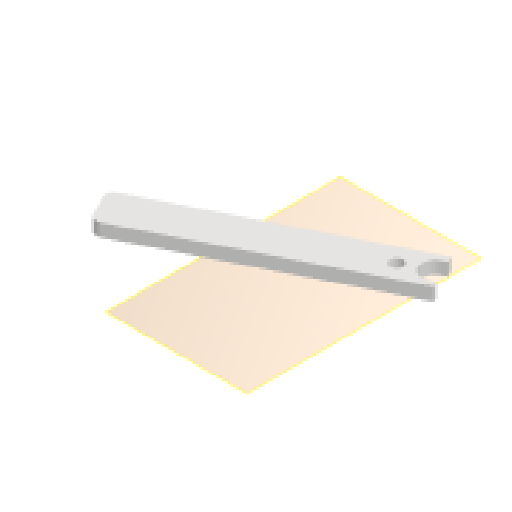
# Autodesk Inventor part: 20_Cube_4_insert_xy_levelarm
Saved by Autodesk Inventor 2025.1 (Build 291241020, 241B)
## iProperties
Created: 2024-10-07
Part Number: 20_Cube_4_insert_xy_levelarm
Material: Generic
Document SubType Name: Modeling
Designer: diederichbenedict
Density: 1 g/cm^3
Appearance: Default
Author: diederichbenedict
Autodesk Inventor part; units mm, degrees
ref_plane "YZ Plane" through (0, 0, 0) normal (1, 0, 0) x (0, 1, 0)
ref_plane "XZ Plane" through (0, 0, 0) normal (0, 1, 0) x (-1, 0, 0)
ref_plane "XY Plane" through (0, 0, 0) normal (0, 0, 1) x (1, 0, 0)
ref_plane "Work Plane1" through (0, 0, 0) normal (0, 0, 1) x (1, 0, 0)
sketch "Sketch1" plane through (0, 0, 0) normal (0, 0, 1) x (1, 0, 0)
  arc A0 (-15, -23) -> (-13.6245, -24.9) centre (-13, -23) ccw projected
  line L0 (-13.6245, -24.9) -> (13.6245, -24.9) projected
  arc A1 (13.6245, -24.9) -> (15, -23) centre (13, -23) ccw projected
  line L1 (15, -23) -> (15, 23) projected
  arc A2 (15, 23) -> (13.6245, 24.9) centre (13, 23) ccw projected
  line L2 (13.6245, 24.9) -> (-13.6245, 24.9) projected
  arc A3 (-13.6245, 24.9) -> (-15, 23) centre (-13, 23) ccw projected
  line L3 (-15, 23) -> (-15, -23) projected
  circle A4 centre (10.5, 13.5) radius 1.4 construction
  circle A5 centre (16.5, 16.5) radius 2.45 projected
  line L4 (-36.2338, -4.8358) -> (15.643, 21.1026)
  line L5 (15.643, 21.1026) -> (19.6679, 13.0528)
  line L6 (19.6679, 13.0528) -> (-32.2089, -12.8856)
  line L7 (-34.8922, -11.9912) -> (-37.1282, -7.519)
  line L8 (-38.0227, -5.7302) -> (19.6679, 13.0528) construction
  line L9 (15.643, 21.1026) -> (-33.9978, -13.78) construction
  line L10 (16.5, 16.5) -> (10.5, 13.5)
  line L11 (16.5, 16.5) -> (19.9213, 18.2106) construction
  line L12 (17.8416, 13.8167) -> (21.2629, 15.5274)
  line L13 (18.5797, 20.8939) -> (15.1584, 19.1833)
  arc A6 (15.1584, 19.1833) -> (17.8416, 13.8167) centre (16.5, 16.5) ccw
  arc A7 (21.2629, 15.5274) -> (18.5797, 20.8939) centre (19.9213, 18.2106) ccw
  arc A8 (-34.8922, -11.9912) -> (-32.2089, -12.8856) centre (-33.1033, -11.0967) ccw
  arc A9 (-36.2338, -4.8358) -> (-37.1282, -7.519) centre (-35.3394, -6.6246) ccw
  circle A10 centre (10.5, 13.5) radius 1.5
  arc A11 (13.5, 9.9688) -> (-21.4758, -7.519) centre (10.6575, -28.0659) ccw
  arc A12 (9.4751, 18.0187) -> (-25.5007, 0.5308) centre (10.6575, -28.0659) ccw
  circle A13 centre (0, -18.9) radius 1.4 projected
  point P0 (0, 0)
  point P1 (-9.1774, 3.6613)
  point P2 (18.2106, 17.3553)
  point P3 (16.3138, 19.761)
  point P4 (18.9971, 14.3944)
  dimension "d0" = 60
  dimension "d1" = 9
  dimension "d2" = 4.5
  dimension "d3" = 8
  dimension "d4" = 6
  dimension "d5" = 2
  dimension "d8" = 3
  dimension "d9" = 14
  dimension "d10" = 14
  constraints: 22 end point, 12 point on circle, 8 point on line, 8 tangent, 7 centre point, 4 parallel, 3 midpoint, 2 coincident, 1 concentric, 1 equal radius, 1 perpendicular
  measures "d0" distance of L8.start L4.end
  measures "d1" distance of L4.end L5.end
  measures "d2" distance from line of A4.centre L6
  measures "d3" distance from line of A4.centre L5
  measures "d4" diameter of A7
  measures "d5" radius of A8
  measures "d8" diameter of A10
  measures "d9" distance from line of L7 A11.end
  measures "d10" distance from line of A12.end L7
extrude "Extrusion1" add sketch "Sketch1" along normal blind 3 contours A11 L6 A8 L7 A9 L4 L3 | L3 L4 L1 A6 L6 A11 | L4 A12 L3 | L3 A12 L4 | L1 A6 L12 L5 L6 | L4 L5 L13 A6 L1
fillet "Fillet1" radius 5 4 edges at (-25.5007, 0.5308, 1.5) (-21.4758, -7.519, 1.5) (9.4751, 18.0187, 1.5) (13.5, 9.9688, 1.5)
sketch "Sketch2" plane through (0, 0, 0) normal (0, 0, -1) x (-1, 0, 0)
  circle A0 centre (-10.5, 13.5) radius 1.1933 projected
  circle A1 centre (-10.5, 13.5) radius 1.5 projected
  circle A2 centre (-10.5, 13.5) radius 3
  point P0 (0, 0)
  dimension "d12" = 6
  constraints: 1 centre point, 1 coincident
  measures "d12" diameter of A2
extrude "Extrusion2" add sketch "Sketch2" along normal blind 0.5 contours A2
body "Solid1"
